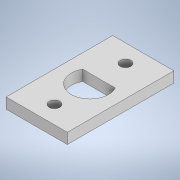
# Autodesk Inventor part: Ответка замка
Saved by Autodesk Inventor 2022 (Build 260153000, 153)
## iProperties
Created: 2025-01-17
Part Number: Ответка замка
Material: Типовые
Document SubType Name: Modeling
Designer: korsh624
Density: 1 g/cm^3
Appearance: По умолчанию
Author: korsh624
Autodesk Inventor part; units mm, degrees
ref_plane "YZ Plane" through (0, 0, 0) normal (1, 0, 0) x (0, 1, 0)
ref_plane "XZ Plane" through (0, 0, 0) normal (0, 1, 0) x (-1, 0, 0)
ref_plane "XY Plane" through (0, 0, 0) normal (0, 0, 1) x (1, 0, 0)
sketch "Эскиз1" plane through (0, 0, 0) normal (0, 1, 0) x (-1, 0, 0)
  arc A0 (4.5891, -2.55) -> (-4.5891, -2.55) centre (0, 0) ccw
  line L0 (4.5891, -2.55) -> (-4.5891, -2.55)
  line L1 (8.5982, 15) -> (-8.6371, 15)
  line L2 (-8.6371, 15) -> (-8.6371, -15)
  line L3 (-8.6371, -15) -> (8.5982, -15)
  line L4 (8.5982, -15) -> (8.5982, 15)
  circle A1 centre (-0.0195, 10) radius 1.5
  circle A2 centre (-0.0195, -10) radius 1.5
  dimension "d0" = 10.5
  dimension "d1" = 2.55
  dimension "d2" = 15
  dimension "d3" = 15
  dimension "d4" = 3
  dimension "d5" = 3
  dimension "d6" = 5
  dimension "d7" = 5
  constraints: 10 end point, 3 centre point, 2 horizontal, 2 parallel, 2 point on circle, 1 coincident, 1 perpendicular
  measures "d0" diameter of A0
  measures "d1" distance from line of L0 A0.centre
  measures "d2" distance from line of L1 A0.centre
  measures "d3" distance from line of L3 point (0, 0)
  measures "d4" diameter of A1
  measures "d5" diameter of A2
  measures "d6" distance from line of A1.centre L1
  measures "d7" distance from line of A2.centre L3
extrude "Выдавливание1" add sketch "Эскиз1" along normal blind 3
